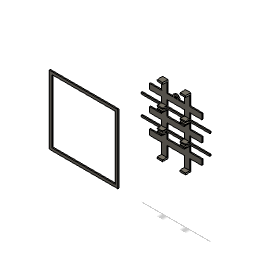
BackPlate_and_Diffuser_Holddown (Autodesk Fusion 360 design; units mm, degrees)
Autodesk Fusion 360 part; units mm, degrees
note: some values were not read from the file. Set by a fixed rule: which sketch regions a step uses.
sketch "Sketch1" plane through (0, 0, 0) normal (0, 0, 1) x (1, 0, 0)
  line L0 (0, 0) -> (128, 0) construction
  line L1 (128, 0) -> (128, 128) construction
  line L2 (128, 128) -> (0, 128) construction
  line L3 (0, 128) -> (0, 0) construction
  line L4 (0, 64) -> (128, 64) construction
  line L5 (64, 128) -> (64, 0) construction
  line L6 (42.6667, 128) -> (42.6667, 0) construction
  line L7 (85.3333, 128) -> (85.3333, 0) construction
  line L8 (128, 101.5) -> (0, 101.5) construction
  line L9 (128, 27.5) -> (0, 27.5) construction
  line L10 (113, 59) -> (15, 59)
  line L11 (15, 59) -> (15, 69)
  line L12 (15, 69) -> (113, 69)
  line L13 (113, 69) -> (113, 59)
  line L14 (113, 59) -> (15, 69) construction
  line L15 (15, 59) -> (113, 69) construction
  line L16 (113, 96.5) -> (15, 96.5)
  line L17 (15, 96.5) -> (15, 106.5)
  line L18 (15, 106.5) -> (113, 106.5)
  line L19 (113, 106.5) -> (113, 96.5)
  line L20 (113, 96.5) -> (15, 106.5) construction
  line L21 (15, 96.5) -> (113, 106.5) construction
  line L22 (113, 22.5) -> (15, 22.5)
  line L23 (15, 22.5) -> (15, 32.5)
  line L24 (15, 32.5) -> (113, 32.5)
  line L25 (113, 32.5) -> (113, 22.5)
  line L26 (113, 22.5) -> (15, 32.5) construction
  line L27 (15, 22.5) -> (113, 32.5) construction
  line L28 (37.6667, 0) -> (47.6667, 0)
  line L29 (47.6667, 0) -> (47.6667, 128)
  line L30 (47.6667, 128) -> (37.6667, 128)
  line L31 (37.6667, 128) -> (37.6667, 0)
  line L32 (37.6667, 0) -> (47.6667, 128) construction
  line L33 (47.6667, 0) -> (37.6667, 128) construction
  line L34 (80.3333, 0) -> (90.3333, 0)
  line L35 (90.3333, 0) -> (90.3333, 128)
  line L36 (90.3333, 128) -> (80.3333, 128)
  line L37 (80.3333, 128) -> (80.3333, 0)
  line L38 (80.3333, 0) -> (90.3333, 128) construction
  line L39 (90.3333, 0) -> (80.3333, 128) construction
  line L40 (0, 83) -> (128, 83) construction
  line L41 (128, 46) -> (0, 46) construction
  line L42 (0, 44.5) -> (128, 44.5)
  line L43 (128, 44.5) -> (128, 47.5)
  line L44 (128, 47.5) -> (0, 47.5)
  line L45 (0, 47.5) -> (0, 44.5)
  line L46 (0, 44.5) -> (128, 47.5) construction
  line L47 (128, 44.5) -> (0, 47.5) construction
  line L48 (0, 81.5) -> (128, 81.5)
  line L49 (128, 81.5) -> (128, 84.5)
  line L50 (128, 84.5) -> (0, 84.5)
  line L51 (0, 84.5) -> (0, 81.5)
  line L52 (0, 81.5) -> (128, 84.5) construction
  line L53 (128, 81.5) -> (0, 84.5) construction
  line L54 (32, 79.5) -> (96, 79.5)
  line L55 (96, 79.5) -> (96, 86.5)
  line L56 (96, 86.5) -> (32, 86.5)
  line L57 (32, 86.5) -> (32, 79.5)
  line L58 (32, 79.5) -> (96, 86.5) construction
  line L59 (96, 79.5) -> (32, 86.5) construction
  line L60 (32, 42.5) -> (96, 42.5)
  line L61 (96, 42.5) -> (96, 49.5)
  line L62 (96, 49.5) -> (32, 49.5)
  line L63 (32, 49.5) -> (32, 42.5)
  line L64 (32, 42.5) -> (96, 49.5) construction
  line L65 (96, 42.5) -> (32, 49.5) construction
  circle A0 centre (64, 107) radius 3
  line L66 (80.3333, 128) -> (47.6667, 128)
  line L67 (47.6667, 128) -> (47.6667, 106.5)
  line L68 (47.6667, 106.5) -> (80.3333, 106.5)
  line L69 (80.3333, 106.5) -> (80.3333, 128)
  circle A1 centre (64, 107) radius 6
  line L70 (37.6667, 128) -> (47.6667, 128)
  line L71 (47.6667, 128) -> (47.6667, 125)
  line L72 (47.6667, 125) -> (37.6667, 125)
  line L73 (37.6667, 125) -> (37.6667, 128)
  line L74 (80.3333, 128) -> (90.3333, 128)
  line L75 (90.3333, 128) -> (90.3333, 125)
  line L76 (90.3333, 125) -> (80.3333, 125)
  line L77 (80.3333, 125) -> (80.3333, 128)
  line L78 (37.6667, 0) -> (47.6667, 0)
  line L79 (47.6667, 0) -> (47.6667, 3)
  line L80 (47.6667, 3) -> (37.6667, 3)
  line L81 (37.6667, 3) -> (37.6667, 0)
  line L82 (80.3333, 0) -> (90.3333, 0)
  line L83 (90.3333, 0) -> (90.3333, 3)
  line L84 (90.3333, 3) -> (80.3333, 3)
  line L85 (80.3333, 3) -> (80.3333, 0)
  point P0 (64, 64)
  point P1 (64, 101.5)
  point P2 (64, 27.5)
  point P3 (42.6667, 64)
  point P4 (85.3333, 64)
  point P5 (64, 46)
  point P6 (64, 83)
  point P7 (64, 83)
  point P8 (64, 46)
  dimension "d22" = 128
  dimension "d23" = 128
  dimension "d24" = 42.6667
  dimension "d25" = 42.6667
  dimension "d30" = 26.5
  dimension "d32" = 100.5
  dimension "d33" = 98
  dimension "d34" = 10
  dimension "d35" = 98
  dimension "d36" = 10
  dimension "d37" = 98
  dimension "d38" = 10
  dimension "d54" = 10
  dimension "d55" = 128
  dimension "d56" = 10
  dimension "d57" = 128
  dimension "d58" = 45
  dimension "d59" = 82
  dimension "d60" = 128
  dimension "d61" = 3
  dimension "d62" = 128
  dimension "d63" = 3
  dimension "d68" = 64
  dimension "d69" = 7
  dimension "d70" = 64
  dimension "d71" = 7
  dimension "d80" = 6
  dimension "d81" = 21
  dimension "d82" = 12
  dimension "d83" = 10
  dimension "d84" = 3
  dimension "d85" = 10
  dimension "d86" = 3
  dimension "d87" = 10
  dimension "d88" = 3
  dimension "d89" = 10
  dimension "d90" = 3
  constraint horizontal L0
  constraint vertical L1
  constraint horizontal L2
  constraint vertical L3
  constraint coincident L0.start L3.end
  constraint midpoint L3 L4.start
  constraint midpoint L1 L4.end
  constraint midpoint L2 L5.start
  constraint midpoint L0 L5.end
  constraint coincident L2 L6.start
  constraint coincident L0 L6.end
  constraint perpendicular L0 L6
  constraint coincident L2 L7.start
  constraint coincident L0 L7.end
  constraint perpendicular L0 L7
  constraint coincident L1 L8.start
  constraint coincident L3 L8.end
  constraint perpendicular L3 L8
  constraint coincident L1 L9.start
  constraint coincident L3 L9.end
  constraint perpendicular L3 L9
  constraint horizontal L10
  constraint perpendicular L10 L11
  constraint parallel L10 L12
  constraint parallel L11 L13
  constraint coincident L14 P0
  constraint coincident L15 P0
  constraint midpoint L4 P0
  constraint horizontal L16
  constraint perpendicular L16 L17
  constraint parallel L16 L18
  constraint parallel L17 L19
  constraint coincident L20 P1
  constraint coincident L21 P1
  constraint midpoint L8 P1
  constraint horizontal L22
  constraint perpendicular L22 L23
  constraint parallel L22 L24
  constraint parallel L23 L25
  constraint coincident L26 P2
  constraint coincident L27 P2
  constraint midpoint L9 P2
  constraint horizontal L28
  constraint perpendicular L28 L29
  constraint parallel L28 L30
  constraint parallel L29 L31
  constraint coincident L32 P3
  constraint coincident L33 P3
  constraint midpoint L6 P3
  constraint horizontal L34
  constraint perpendicular L34 L35
  constraint parallel L34 L36
  constraint parallel L35 L37
  constraint coincident L38 P4
  constraint coincident L39 P4
  constraint midpoint L7 P4
  constraint coincident L3 L40.start
  constraint coincident L1 L40.end
  constraint perpendicular L1 L40
  constraint coincident L1 L41.start
  constraint perpendicular L1 L41
  constraint coincident L3 L41.end
  constraint horizontal L42
  constraint perpendicular L42 L43
  constraint parallel L42 L44
  constraint parallel L43 L45
  constraint coincident L46 P8
  constraint coincident L47 P8
  constraint midpoint L41 P8
  constraint horizontal L48
  constraint perpendicular L48 L49
  constraint parallel L48 L50
  constraint parallel L49 L51
  constraint coincident L52 P7
  constraint coincident L53 P7
  constraint midpoint L40 P7
  constraint horizontal L54
  constraint perpendicular L54 L55
  constraint parallel L54 L56
  constraint parallel L55 L57
  constraint coincident L58 P7
  constraint coincident L59 P7
  constraint coincident P7 P6
  constraint horizontal L60
  constraint perpendicular L60 L61
  constraint parallel L60 L62
  constraint parallel L61 L63
  constraint coincident L64 P8
  constraint coincident L65 P8
  constraint coincident P8 P5
  constraint coincident L5 A0.centre
  constraint horizontal L66
  constraint vertical L67
  constraint horizontal L68
  constraint vertical L69
  constraint coincident L18 L67.end
  constraint coincident L29 L67.end
  constraint concentric A0 A1
  constraint horizontal L70
  constraint vertical L71
  constraint horizontal L72
  constraint vertical L73
  constraint horizontal L74
  constraint vertical L75
  constraint horizontal L76
  constraint vertical L77
  constraint horizontal L78
  constraint vertical L79
  constraint horizontal L80
  constraint vertical L81
  constraint horizontal L82
  constraint vertical L83
  constraint horizontal L84
  constraint vertical L85
  measures "d22" distance of L0.start L0.end
  measures "d23" distance of L0.start L2.end
  measures "d24" distance of L3 L6
  measures "d25" distance of L1 L7
  measures "d30" distance of L2 L8
  measures "d32" distance of L2 L9
  measures "d33" distance of L11.end L12.end
  measures "d34" distance of L10.end L11.end
  measures "d35" distance of L17.end L18.end
  measures "d36" distance of L16.end L17.end
  measures "d37" distance of L23.end L24.end
  measures "d38" distance of L22.end L23.end
  measures "d54" distance of L29.end L30.end
  measures "d55" distance of L28.end L29.end
  measures "d56" distance of L35.end L36.end
  measures "d57" distance of L34.end L35.end
  measures "d58" distance of L2 L40
  measures "d59" distance of L2 L41
  measures "d60" distance of L43.end L44.end
  measures "d61" distance of L42.end L43.end
  measures "d62" distance of L49.end L50.end
  measures "d63" distance of L48.end L49.end
  measures "d68" distance of L55.end L56.end
  measures "d69" distance of L54.end L55.end
  measures "d70" distance of L61.end L62.end
  measures "d71" distance of L60.end L61.end
  measures "d80" diameter of A0
  measures "d81" distance of L2 A0.centre
  measures "d82" diameter of A1
  measures "d83" distance of L30.end L29.end
  measures "d84" distance of L30.end L72.end
  measures "d85" distance of L36.end L35.end
  measures "d86" distance of L36.end L76.end
  measures "d87" distance of L28.start L28.end
  measures "d88" distance of L28.start L80.end
  measures "d89" distance of L34.start L34.end
  measures "d90" distance of L34.start L84.end
extrude "Extrude5" add sketch "Sketch1" along normal blind 2 contours L10 L12 L13 L35 | L10 L35 L37 L62 | L10 L12 L35 L37 | L10 L12 L29 L37 | L35 L37 L44 L62 | L12 L35 L37 L54 | L10 L29 L31 L62 | L10 L12 L29 L31 | L35 L42 L44 L61 | L35 L37 L42 L44 | L35 L37 L48 L54 | L10 L11 L12 L31 | L29 L31 L44 L62 | L12 L29 L31 L54 | L29 L37 L42 L44 | L35 L37 L42 L60 | L42 L43 L44 L61 | L35 L37 L48 L50 | L35 L48 L50 L55 | L29 L31 L42 L44 | L29 L31 L48 L54 | L29 L37 L48 L50 | L24 L35 L37 L60 | L35 L37 L50 L56 | L48 L49 L50 L55 | L31 L42 L44 L63 | L29 L31 L42 L60 | L29 L31 L48 L50 | L22 L24 L35 L37 | L22 L24 L25 L35 | L16 L35 L37 L56 | L31 L48 L50 L57 | L42 L44 L45 L63 | L24 L29 L31 L60 | L29 L31 L50 L56 | L22 L24 L29 L37 | L22 L35 L37 L84 | L16 L18 L19 L35 | L16 L18 L35 L37 | L48 L50 L51 L57 | L22 L24 L29 L31 | L16 L29 L31 L56 | L16 L18 L29 L37 L68 A1 | L34 L35 L37 L82 L83 L84 L85 | L18 L35 L37 L69 L76 | L22 L23 L24 L31 | L22 L29 L31 L80 | L16 L18 L29 L31 | L35 L36 L37 L69 L74 L75 L76 L77 | L16 L17 L18 L31 | L28 L29 L31 L78 L79 L80 L81 | L18 L29 L31 L67 L72 | L18 A0 L68 A1 | L18 A0 L68 A1 | L29 L30 L31 L67 L70 L71 L72 L73 | L18 A0 L68 picked at (64.2198, 105.6911) makes body 1
extrude "Extrude6" add sketch "Sketch1" along normal blind 10 contours L35 L37 L44 L62 | L35 L37 L48 L54 | L29 L31 L44 L62 | L35 L37 L42 L60 | L29 L31 L48 L54 | L35 L37 L50 L56 | L29 L31 L42 L60 | L29 L31 L50 L56 bodies 1
extrude "Extrude7" add sketch "Sketch1" along normal blind 10 contours L34 L35 L37 L82 L83 L84 L85 | L35 L36 L37 L69 L74 L75 L76 L77 | L28 L29 L31 L78 L79 L80 L81 | L29 L30 L31 L67 L70 L71 L72 L73 bodies 1
sketch "Sketch2" plane through (0, 0, 0) normal (0, 0, 1) x (1, 0, 0)
  line L0 (-43.909, -93.4786) -> (-171.909, -93.4786)
  line L1 (-171.909, -93.4786) -> (-171.909, 34.5214)
  line L2 (-171.909, 34.5214) -> (-43.909, 34.5214)
  line L3 (-43.909, 34.5214) -> (-43.909, -93.4786)
  line L4 (-43.909, -93.4786) -> (-171.909, 34.5214) construction
  line L5 (-171.909, -93.4786) -> (-43.909, 34.5214) construction
  line L6 (-48.909, -88.4786) -> (-166.909, -88.4786)
  line L7 (-166.909, -88.4786) -> (-166.909, 29.5214)
  line L8 (-166.909, 29.5214) -> (-48.909, 29.5214)
  line L9 (-48.909, 29.5214) -> (-48.909, -88.4786)
  line L10 (-48.909, -88.4786) -> (-166.909, 29.5214) construction
  line L11 (-166.909, -88.4786) -> (-48.909, 29.5214) construction
  point P0 (-107.909, -29.4786)
  point P1 (-107.909, -29.4786)
  dimension "d93" = 128
  dimension "d94" = 128
  dimension "d95" = 118
  dimension "d96" = 118
  constraint horizontal L0
  constraint perpendicular L0 L1
  constraint parallel L0 L2
  constraint parallel L1 L3
  constraint coincident L4 P1
  constraint coincident L5 P1
  constraint horizontal L6
  constraint perpendicular L6 L7
  constraint parallel L6 L8
  constraint parallel L7 L9
  constraint coincident L10 P1
  constraint coincident L11 P1
  constraint coincident P1 P0
  measures "d93" distance of L1.end L2.end
  measures "d94" distance of L0.end L1.end
  measures "d95" distance of L7.end L8.end
  measures "d96" distance of L6.end L7.end
extrude "Extrude8" add sketch "Sketch2" along normal blind 2 separate body makes body 2
equation "BoxInner = 128 mm"
equation "RailWidth = 10 mm"
equation "RailSeparation = ( BoxInner - ( RailWidth * 2 ) ) / 3"
equation "LedLength = 98 mm"
equation "PanelThickness = 3 mm"
equation "d22 = BoxInner"
equation "d23 = BoxInner"
equation "d24 = BoxInner / 3"
equation "d25 = BoxInner / 3"
equation "d30 = R_Horizontal"
equation "d32 = P_Horizontal"
equation "d33 = LedLength"
equation "d34 = RailWidth"
equation "d35 = LedLength"
equation "d36 = RailWidth"
equation "d37 = LedLength"
equation "d38 = RailWidth"
equation "RailEdge = 2 mm"
equation "Thickness = 2 mm"
equation "Depth = 59 mm"
equation "d54 = RailWidth"
equation "d55 = BoxInner"
equation "d56 = RailWidth"
equation "d57 = BoxInner"
equation "d58 = RM_Horizontal"
equation "d59 = MP_Horizontal"
equation "d60 = BoxInner"
equation "d61 = PanelThickness"
equation "d62 = BoxInner"
equation "d63 = PanelThickness"
equation "d68 = BoxInner / 2"
equation "d69 = PanelThickness + RailEdge * 2"
equation "d70 = BoxInner / 2"
equation "d71 = PanelThickness + RailEdge * 2"
equation "d72 = Thickness"
equation "d74 = Thickness * 5"
equation "R_Horizontal = 26.5 mm"
equation "RM_Horizontal = 45 mm"
equation "MP_Horizontal = 82 mm"
equation "P_Horizontal = 100.5 mm"
equation "d83 = RailWidth"
equation "d84 = PanelThickness"
equation "d85 = RailWidth"
equation "d86 = PanelThickness"
equation "d87 = RailWidth"
equation "d88 = PanelThickness"
equation "d89 = RailWidth"
equation "d90 = PanelThickness"
